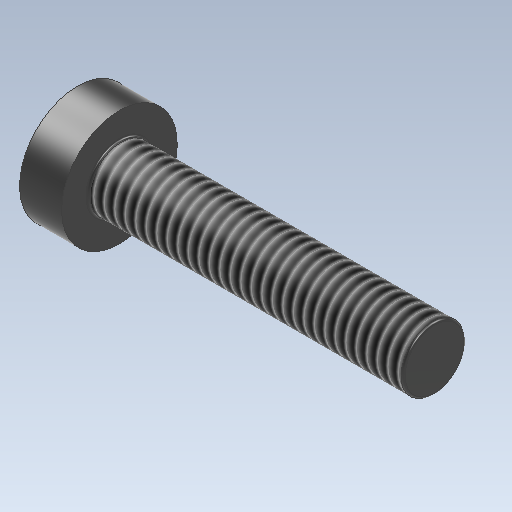
# Autodesk Inventor part: ネジキャップM3L15
Saved by Autodesk Inventor 2020.2 (Build 242310000, 310)
## iProperties
Created: 2020-02-24
Part Number: ネジキャップM3L15
Material: 鋼
Document SubType Name: Modeling
Designer: aoyam
Density: 7.85 g/cm^3
Appearance: サテン - 黒
Mass: 0.577682 g
Surface Area: 1.30939 cm^2
Volume: 0.0735901 cm^3
Author: aoyam
Autodesk Inventor part; units mm, degrees
ref_plane "YZ Plane" through (0, 0, 0) normal (1, 0, 0) x (0, 1, 0)
ref_plane "XZ Plane" through (0, 0, 0) normal (0, 1, 0) x (-1, 0, 0)
ref_plane "XY Plane" through (0, 0, 0) normal (0, 0, 1) x (1, 0, 0)
sketch "スケッチ1" plane through (0, 0, 0) normal (0, 0, 1) x (1, 0, 0)
  line L0 (0, 0) -> (15, 0)
  line L1 (15, 0) -> (15, 1.5)
  line L2 (15, 1.5) -> (0, 1.5)
  line L3 (0, 1.5) -> (0, 0)
  line L4 (0, 0) -> (0, 2.75)
  line L5 (0, 0) -> (-2, 0)
  line L6 (-2, 0) -> (0, 0)
  line L7 (-2, 0) -> (-2, 1.15)
  line L8 (0, 0) -> (-2, 0)
  line L9 (-2, 0) -> (-2, 2.75)
  line L10 (-2, 2.75) -> (0, 2.75)
  line L11 (0, 2.75) -> (0, 0)
  dimension "d0" = 1.5
  dimension "d1" = 15
  dimension "d3" = 2
  dimension "d4" = 2.75
  dimension "d5" = 1.15
  constraints: 24 end point, 4 parallel, 3 horizontal, 2 perpendicular, 2 vertical
  measures "d0" distance of L1.end L0.end
  measures "d1" distance of L1.end L2.end
  measures "d3" distance of L0.start L5.end
  measures "d4" distance of L0.start L4.end
  measures "d5" distance of L5.end L7.end
revolve "回転1" add sketch "スケッチ1" angle 360 about axis through (-2, 0, 0) along (1, 0, 0)
thread "ねじ1" size "M3x0.5" class "6g" standard "ANSI Metric M Profile" length 100
sketch "スケッチ2" plane through (-2, 0, 0) normal (-1, 0, 0) x (0, 0, 1)
  line L0 (-0.575, 0.9959) -> (0.575, 0.9959)
  line L1 (0.575, 0.9959) -> (1.15, 0)
  line L2 (1.15, 0) -> (0.575, -0.9959)
  line L3 (0.575, -0.9959) -> (-0.575, -0.9959)
  line L4 (-0.575, -0.9959) -> (-1.15, 0)
  line L5 (-1.15, 0) -> (-0.575, 0.9959)
  point P0 (0, 0)
  point P1 (0, 0)
  point P2 (0, 0)
  dimension "d10" = 1.15
  dimension "d11" = 1.9919
  constraints: 12 end point, 1 coincident, 1 horizontal, 13 other
  measures "d10" distance of L0.start L0.end
  measures "d11" distance between parallel lines of L3 L0
extrude "押し出し1" cut sketch "スケッチ2" against normal blind 1.4
fillet "フィレット1" radius 0.2 6 edges at (-0.6, 0.9959, 0) (-0.6, 0.498, 0.8625) (-0.6, 0.498, -0.8625) (-0.6, -0.498, -0.8625) (-0.6, -0.9959, 0) (-0.6, -0.498, 0.8625)
fillet "フィレット2" radius 0.1 1 edges at (0, -1.5, 0)
fillet "フィレット3" radius 0.1 1 edges at (15, -1.5, 0)
